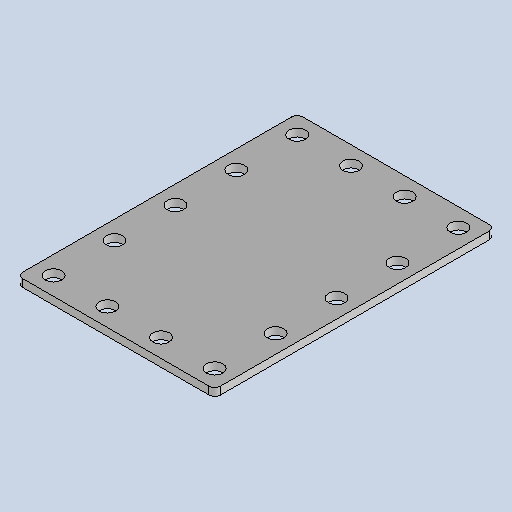
# Autodesk Inventor part: PRS 9607 charging flange rect_D1200 940
Saved by Autodesk Inventor 2026.2 (Build 302298010, 298A)
## iProperties
Created: 2025-02-13
Part Number: PRS 9607 charging flange rect_D1200 940
Material: Steel
Document SubType Name: Sheet Metal
Designer: admin
Mass: 3436.88 g
Surface Area: 1231.62 cm^2
Volume: 437.819 cm^3
Density: 7.85 g/cm^3
Flat Pattern Width: 29.2 cm
Flat Pattern Length: 20.6 cm
Flat Pattern Area: 601.52 cm^2
Sheet Metal Rule: AISI304 4mm Die 32
Sheet Metal Width: 292,000 mm
Sheet Metal Length: 206,000 mm
Sheet Metal Area: 60152,000 mm^2
Appearance: Default
Author: pokla
Autodesk Inventor part; units mm, degrees
ref_plane "YZ Plane" through (0, 0, 0) normal (1, 0, 0) x (0, 1, 0)
ref_plane "XZ Plane" through (0, 0, 0) normal (0, 1, 0) x (-1, 0, 0)
ref_plane "XY Plane" through (0, 0, 0) normal (0, 0, 1) x (1, 0, 0)
sketch "Sketch2" plane through (0, 0, 0) normal (0, 0, 1) x (1, 0, 0)
  line L0 (-53, -96) -> (53, -96)
  line L1 (53, -96) -> (53, 96)
  line L2 (53, 96) -> (-53, 96)
  line L3 (-53, 96) -> (-53, -96)
  line L4 (-53, -96) -> (53, 96) construction
  line L5 (53, -96) -> (-53, 96) construction
  line L6 (-103, -146) -> (103, -146)
  line L7 (103, -146) -> (103, 146)
  line L8 (103, 146) -> (-103, 146)
  line L9 (-103, 146) -> (-103, -146)
  point P0 (0, 0)
  dimension "d31" = 50
  dimension "d60" = 192
  dimension "d61" = 106
  measures "d31" distance between parallel lines of L3 L9
  measures "d60" distance of L2.end L0.start
  measures "d61" distance of L0.start L0.end
extrude "Plate2" add sketch "Sketch2" along normal blind 8 contours L3 L2 L1 L0 | L9 L8 L7 L6
sketch "Sketch5" plane through (0, 0, 8) normal (0, 0, 1) x (1, 0, 0)
  line L0 (103, -146) -> (-103, -146) construction
  line L1 (103, 146) -> (103, -146) construction
  line L2 (-103, 146) -> (103, 146) construction
  line L3 (-103, -146) -> (-103, 146) construction
  line L4 (-84, 127) -> (84, 127) construction
  line L5 (84, 127) -> (84, -127) construction
  line L6 (84, -127) -> (-84, -127) construction
  line L7 (-84, -127) -> (-84, 127) construction
  line L8 (-28, -127) -> (28, -127)
  line L9 (28, -127) -> (28, 127) construction
  line L10 (28, 127) -> (-28, 127)
  line L11 (-28, 127) -> (-28, -127) construction
  line L12 (-28, 0) -> (28, 0) construction
  point P0 (0, 0)
  point P1 (0, -127)
  point P2 (-84, -63.5)
  point P3 (-84, 0)
  point P4 (-84, 63.5)
  point P5 (84, 63.5)
  point P6 (84, 0)
  point P7 (84, -63.5)
  point P8 (0, 0)
  dimension "d34" = 19
  dimension "d47" = 63.5
  dimension "d48" = 63.5
  dimension "d49" = 56
  dimension "d50" = 56
  constraints: 18 end point, 8 point on line, 6 midpoint, 5 coincident, 2 parallel, 2 symmetric about line, 1 horizontal, 1 horizontal alignment, 1 perpendicular, 3 other
  measures "d34" distance between parallel lines of L0 L6
  measures "d47" distance of point (-84, -63.5) point (-84, -127)
  measures "d48" distance of point (-84, 0) point (-84, -63.5)
  measures "d49" distance of L8.start point (-84, -127)
  measures "d50" distance of L8.end L8.start
fillet "Corner Round1" radius 6 4 edges at (-103, -146, 4) (-103, 146, 4) (103, 146, 4) (103, -146, 4)
hole "Hole1" at (-84, -127, 8) at (-84, -63.5, 8) at (-84, 0, 8) at (-84, 63.5, 8) at (-84, 127, 8) at (84, 127, 8) at (84, 63.5, 8) at (84, 0, 8) at (84, -63.5, 8) at (84, -127, 8) at (-28, -127, 8) at (28, 127, 8) at (28, -127, 8) at (-28, 127, 8) direction (0, 0, -1) diameter 17 end through all
equation "\"d47\" = d48"
equation "\"d49\" = d50"
equation "\"d60\" = ChargingHatch_width - 2 * Thickness"
equation "\"d61\" = ChargingHatch_hight - 2 * Thickness"
equation "\"d56\" = Thickness"
equation "\"d14\" = Thickness"
equation "\"BendReliefWidth\" = Thickness"
equation "\"BendReliefDepth\" = 0.5 * Thickness"
equation "\"CornerReliefSize\" = 4 * Thickness"
equation "\"MinimumRemnant\" = 2 * Thickness"
equation "\"TransitionRadius\" = BendRadius"
equation "\"JacobiRadiusSize\" = BendRadius"
equation "\"GapSize\" = Thickness"
equation "\"ChargingHatch_width\" = 208"
equation "\"Thickness\" = 8"
equation "\"ChargingHatch_hight\" = 122"
equation "\"BendRadius\" = 6"
body "Solid3"
